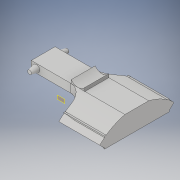
# Autodesk Inventor part: index_clamp
Saved by Autodesk Inventor 2018 (Build 220112000, 112)
## iProperties
Created: 2018-03-09
Part Number: index_clamp
Material: Generic
Document SubType Name: Modeling
Designer: rheal
Density: 1 g/cm^3
Appearance: Default
Author: rheal
Autodesk Inventor part; units mm, degrees
ref_plane "YZ Plane" through (0, 0, 0) normal (1, 0, 0) x (0, 1, 0)
ref_plane "XZ Plane" through (0, 0, 0) normal (0, 1, 0) x (-1, 0, 0)
ref_plane "XY Plane" through (0, 0, 0) normal (0, 0, 1) x (1, 0, 0)
sketch "Sketch1" plane through (0, 0, 0) normal (0, 1, 0) x (-1, 0, 0)
  line L0 (-13.75, 3.5) -> (13.75, 3.5)
  line L1 (13.75, 3.5) -> (13.75, -3.5)
  line L2 (13.75, -3.5) -> (-13.75, -3.5)
  line L3 (-13.75, -3.5) -> (-13.75, 3.5)
  line L4 (-13.75, 3.5) -> (13.75, -3.5) construction
  line L5 (13.75, 3.5) -> (-13.75, -3.5) construction
  point P0 (0, 0)
  dimension "d0" = 27.5
  dimension "d1" = 7
  constraints: 12 end point, 2 midpoint, 2 parallel, 1 horizontal, 1 perpendicular
  measures "d0" distance of L1.end L2.end
  measures "d1" distance of L0.end L1.end
extrude "Extrusion1" add sketch "Sketch1" along normal blind 2.5
sketch "Sketch2" plane through (13.75, 0, -3.5) normal (0, 0, -1) x (-1, 0, 0)
  line L0 (27.5, 0) -> (27.5, 2.5) projected
  line L1 (27.5, 1.25) -> (26, 1.25)
  circle A0 centre (26, 1.25) radius 1
  point P0 (13.75, 0)
  dimension "d4" = 1.5
  dimension "d5" = 2
  constraints: 2 end point, 1 centre point, 1 coincident, 1 horizontal, 1 midpoint
  measures "d4" distance of L1.start L1.end
  measures "d5" diameter of A0
extrude "Extrusion2" add sketch "Sketch2" along normal blind 2 draft -12
sketch "Sketch3" plane through (13.75, 0, 3.5) normal (1, 0, 0) x (0, 0, -1)
  line L0 (0, 2.5) -> (7, 2.5) projected
  line L1 (3.5, 2.5) -> (3.5, -12.5)
  line L2 (7, 0) -> (7, 2.5) projected
  arc A0 (14.3915, -1.6085) -> (7, 2.5) centre (3.5, -12.5) ccw
  arc A1 (12.6788, -3.3212) -> (3.5, 0.4808) centre (3.5, -12.5) ccw
  line L3 (3.5, -12.5) -> (14.3915, -1.6085)
  line L4 (3.5, -12.5) -> (18.9029, -12.5) construction
  line L5 (7, 0) -> (7, 2.5)
  point P0 (3.5, 0)
  dimension "d8" = 15
  dimension "d9" = 45
  constraints: 8 end point, 6 point on circle, 3 point on line, 2 centre point, 2 coincident, 2 vertical, 1 equal length, 1 horizontal, 1 midpoint
  measures "d8" distance of L1.start L1.end
  measures "d9" angle of L4 L3
extrude "Extrusion3" add sketch "Sketch3" against normal blind 12 contours L0 L2 A1 L1 | A0 L3 A1 L2
sketch "Sketch4" plane through (-13.75, 0, 3.5) normal (0, 0, 1) x (1, 0, 0)
  line L0 (0, 2.5) -> (27.5, 2.5) projected
  line L1 (13.75, 2.5) -> (15.75, 2.5)
  line L2 (15.75, 2.5) -> (11.75, 2.5)
  line L3 (11.75, 2.5) -> (11.75, 3.5)
  line L4 (11.75, 3.5) -> (15.75, 3.5)
  line L5 (15.75, 3.5) -> (15.75, 2.5)
  arc A0 (11.75, 3.5) -> (15.75, 3.5) centre (13.75, 5) ccw
  point P0 (13.75, 0)
  dimension "d12" = 2
  dimension "d13" = 4
  dimension "d14" = 1
  constraints: 10 end point, 3 perpendicular, 3 point on circle, 2 point on line, 1 centre point, 1 midpoint
  measures "d12" distance of L1.start L1.end
  measures "d13" distance of L1.end L2.end
  measures "d14" distance of L2.end L3.end
extrude "Extrusion4" add sketch "Sketch4" against normal blind 3.5 contours L3 A0 L0 | A0 L5 L0
fillet "Fillet1" radius 4 1 edges at (1.75, 1.25, -3.5)
mirror "Mirror1" about plane through (1.2398, 2.7314, 0) normal (0, 0, -1)
ref_plane "Work Plane1" through (2, 2.5, 9.5) normal (0, 0, 1) x (1, 0, 0)
sketch "Sketch6" plane through (2, 2.5, 9.5) normal (0, 0, 1) x (1, 0, 0)
  line L0 (11.75, -2.5) -> (11.75, -5.8212) projected
  line L1 (11.75, -5.8894) -> (11.75, -2.5)
  line L2 (-4.25, -2.5) -> (11.75, -2.5) projected
  line L3 (11.75, -2.5) -> (-0.25, -2.5)
  arc A0 (11.75, -5.8212) -> (-0.25, -2.5) centre (-2.078, -32.4443) ccw
  point P0 (-2, -2.5)
  dimension "d25" = 12
  dimension "d26" = 30
  constraints: 4 end point, 2 point on circle, 1 centre point, 1 collinear, 1 point on line
  measures "d25" distance of L0.start L3.end
  measures "d26" radius of A0
extrude "Extrusion6" add sketch "Sketch6" against normal blind 19
body "Solid1"
